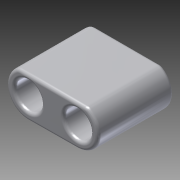
# Autodesk Inventor part: link_joint_v5_z15_Dr1.5
Saved by Autodesk Inventor 2015 (Build 190159000, 159)
## iProperties
Created: 2016-02-21
Part Number: link_joint_v5_z15_Dr1.5
Material: Plástico ABS
Document SubType Name: Modeling
Designer: JavierPC
Density: 1.06 g/cm^3
Appearance: Suave - Blanco
Author: JavierPC
Autodesk Inventor part; units mm, degrees
ref_plane "YZ Plane" through (0, 0, 0) normal (1, 0, 0) x (0, 1, 0)
ref_plane "XZ Plane" through (0, 0, 0) normal (0, 1, 0) x (-1, 0, 0)
ref_plane "XY Plane" through (0, 0, 0) normal (0, 0, 1) x (1, 0, 0)
sketch "Boceto6" plane through (0, 0, 0) normal (0, 1, 0) x (-1, 0, 0)
  line L0 (-120.9824, 0) -> (124.9062, 0)
  line L1 (-0.0006, 74.2244) -> (-0.0006, -71.6145)
  line L2 (-0.0006, 74.2244) -> (145.8383, 74.2244) construction
  circle A0 centre (-1.56, 0) radius 0.85
  circle A1 centre (1.5587, 0) radius 0.85
  line L3 (-1.5578, 1.3336) -> (1.5475, 1.3593)
  line L4 (-1.5578, -1.3336) -> (1.5475, -1.3593)
  arc A2 (-1.5578, 1.3336) -> (-1.5578, -1.3336) centre (-1.56, 0) ccw
  arc A3 (1.5475, -1.3593) -> (1.5475, 1.3593) centre (1.5587, 0) ccw
  point P0 (0, 0)
  dimension "d22" = 90
  dimension "d23" = 1.7
  dimension "d24" = 1.7
  dimension "d25" = 3.1187
  dimension "d26" = 3.1187
  dimension "d34" = 1.3593
  constraints: 10 end point, 4 centre point, 4 point on circle, 3 horizontal, 2 coincident, 2 point on line, 2 tangent, 1 perpendicular
  measures "d22" angle of L1 L2
  measures "d23" diameter of A0
  measures "d24" diameter of A1
  measures "d25" distance of A1.centre A0.centre
  measures "d26" diameter of A0.centre L1
  measures "d34" radius of A3
extrude "Extrusión6" add sketch "Boceto6" along normal mid plane 4.8 contours A2 L3 L1 L0 A0 | L0 A0 L1 L4 A2 | L3 A3 L0 A1 L1 | L1 L0 A1 A3 L4
sketch "Boceto7" plane through (0, 0, 0) normal (0, 1, 0) x (-1, 0, 0)
  line L0 (4.4458, 2.3025) -> (-3.9017, 2.3025)
  line L1 (-3.9017, 2.3025) -> (-3.9017, 1.2)
  line L2 (-3.9017, 1.2) -> (4.4458, 1.2)
  line L3 (4.4458, 1.2) -> (4.4458, 2.3025)
  circle A0 centre (-1.56, 0) radius 0.85 projected
  point P0 (0, 0)
  dimension "d35" = 1.2
  constraints: 8 end point, 2 parallel, 1 horizontal, 1 perpendicular
  measures "d35" distance from line of A0.centre L2
extrude "Extrusión7" cut sketch "Boceto7" along normal mid plane 10 contours L3 L2 L1 L0
fillet "Empalme2" radius 0.2 4 edges at (-0.7087, -2.4, 0) (-0.7087, 2.4, 0) (2.41, -2.4, 0) (2.41, 2.4, 0)
fillet "Empalme2" radius 0.2 8 edges at (-0.0278, -2.4, 1.2) (-2.8763, -2.4, -0.3345) (0.0051, -2.4, -1.3465) (2.8595, -2.4, -0.2996) (-0.0278, 2.4, 1.2) (2.8595, 2.4, -0.2996) (0.0051, 2.4, -1.3465) (-2.8763, 2.4, -0.3345)
fillet "Empalme2" radius 0.5 2 edges at (-2.1973, 0, 1.2) (2.1418, 0, 1.2)
equation "\"d25\" = p"
equation "\"d26\" = p"
equation "\"Dp\" = 15"
equation "\"p\" = 3.118675"
